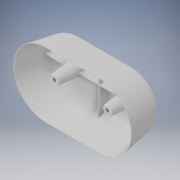
# Autodesk Inventor part: Součást11
Saved by Autodesk Inventor 2019 (Build 230136000, 136)
## iProperties
Created: 2019-11-19
Part Number: Součást11
Material: Všeobecné
Document SubType Name: Modeling
Designer: hynek
Density: 1 g/cm^3
Appearance: Výchozí
Author: hynek
Autodesk Inventor part; units mm, degrees
ref_plane "YZ Plane" through (0, 0, 0) normal (1, 0, 0) x (0, 1, 0)
ref_plane "XZ Plane" through (0, 0, 0) normal (0, 1, 0) x (-1, 0, 0)
sketch "Náčrt1" plane through (0, 0, 0) normal (0, 0, 1) x (1, 0, 0)
  line L0 (-168, 0) -> (168, 0) construction
  line L1 (0, -84) -> (0, 84) construction
  arc A0 (-60, 60) -> (-60, -60) centre (-60, 0) ccw
  line L2 (-60, 60) -> (0, 60)
  line L3 (-60, -60) -> (0, -60)
  arc A1 (60, -60) -> (60, 60) centre (60, 0) ccw
  line L4 (60, 60) -> (0, 60)
  line L5 (60, -60) -> (0, -60)
  point P0 (0, 0)
  dimension "d0" = 60
  constraints: 8 end point, 4 point on circle, 3 point on line, 3 symmetric about line, 3 tangent, 2 centre point, 2 perpendicular, 1 midpoint, 1 other
  measures "d0" radius of A0
extrude "Vysunutí1" add sketch "Náčrt1" along normal blind 80 draft 10
fillet "Zaoblení1" radius 20 6 edges at (120, 0, 0) (-30, 60, 0) (30, 60, 0) (-120, 0, 0) (30, -60, 0) (-30, -60, 0)
shell "Skořepina1" thickness 1 removed faces 1 at (-40, -24.7021, 80)
sketch "Náčrt2" plane through (-60, 43.218, 1) normal (0, 0, 1) x (1, 0, 0)
  arc A0 (0, 0) -> (0, -86.436) centre (0, -43.218) ccw projected
  circle A1 centre (0, -43.218) radius 17
  point P0 (60, -43.218)
  dimension "d5" = 34
  constraints: 1 centre point, 1 coincident
  measures "d5" diameter of A1
extrude "Vysunutí2" add sketch "Náčrt2" along normal blind 60 draft -6
sketch "Náčrt3" plane through (0, 0, 0) normal (0, 0, -1) x (-1, 0, 0)
  circle A0 centre (60, 0) radius 17 construction
  circle A1 centre (60, 0) radius 16
  point P0 (0, 0)
  dimension "d8" = 1
  constraints: 1 centre point, 1 coincident
  measures "d8" radial gap between concentric circles of A0 A1
extrude "Vysunutí3" cut sketch "Náčrt3" against normal blind 60 draft -6
fillet "Zaoblení2" radius 6 1 edges at (-77, 0, 1)
fillet "Zaoblení2" radius 5 1 edges at (-44, 0, 0)
fillet "Zaoblení3" radius 2 1 edges at (-50.3063, 0, 60)
fillet "Zaoblení3" radius 3 1 edges at (-70.6937, 0, 61)
sketch "Náčrt4" plane through (-60, 0, 61) normal (0, 0, 1) x (1, 0, 0)
  circle A0 centre (0, 0) radius 7.9925 construction
  point P0 (60, 0)
hole "Díra1" at (-60, 0, 61) direction (0, 0, -1) diameter 8 end through all
mirror "Zrcadlit1" about plane through (0, 0, 0) normal (1, 0, 0) of "Vysunutí2", "Vysunutí3", "Zaoblení2", "Zaoblení3", "Díra1"
ref_plane "Pracovní rovina1" through (0, 0, 20) normal (0, 0, 1) x (1, 0, 0)
sketch "Náčrt5" plane through (0, 0, 20) normal (0, 0, 1) x (1, 0, 0)
  circle A0 centre (60, 0) radius 15.003 construction
  circle A1 centre (60, 0) radius 13.8979 construction
  circle A2 centre (-60, 0) radius 15.003 construction
  circle A3 centre (-60, 0) radius 13.8979 construction
  line L0 (-60, -62.5111) -> (60, -62.5111) construction
  arc A4 (60, -62.5111) -> (60, 62.5111) centre (60, 0) ccw construction
  line L1 (60, 62.5111) -> (-60, 62.5111) construction
  arc A5 (-60, 62.5111) -> (-60, -62.5111) centre (-60, 0) ccw construction
  line L2 (60, -63.5265) -> (-60, -63.5265) construction
  arc A6 (-60, 63.5265) -> (-60, -63.5265) centre (-60, 0) ccw construction
  line L3 (-60, 63.5265) -> (60, 63.5265) construction
  arc A7 (60, -63.5265) -> (60, 63.5265) centre (60, 0) ccw construction
  line L4 (-187.7486, 0) -> (187.7486, 0) construction
  line L5 (0, -103.7486) -> (0, 103.7486) construction
  arc A8 (-60, 61.9294) -> (-60, -61.9294) centre (-60, 0) ccw projected
  line L6 (-121.9294, 0) -> (-80.502, 0)
  circle A9 centre (-60, 0) radius 20.502 projected
  line L7 (-37.7869, 0) -> (39.498, 0)
  circle A10 centre (60, 0) radius 20.502 projected
  line L8 (82.2082, 0) -> (123.5265, 0)
  line L9 (-60, 62.9142) -> (60, 62.9142) projected
  line L10 (0, 62.9142) -> (0, -63.5265)
  point P0 (0, 0)
  constraints: 8 end point, 2 horizontal alignment, 2 midpoint, 2 point on circle, 1 point on line, 9 other
rib "Žebro1" sketch "Náčrt5" thickness 2 direction (0, 0, -1) end up to next extend profile yes curves L6 L7 L10 L8
